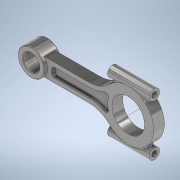
# Autodesk Inventor part: connecting_rod
Saved by Autodesk Inventor 2021 (Build 250183000, 183)
## iProperties
Created: 2020-11-10
Part Number: connecting_rod
Material: Сталь, высокопрочная, низколегированная
Document SubType Name: Modeling
Designer: panda
Density: 7.85 g/cm^3
Appearance: Сталь — полированная
Mass: 1160.23 g
Surface Area: 416.927 cm^2
Volume: 147.8 cm^3
Author: panda
Autodesk Inventor part; units mm, degrees
ref_plane "XZ Plane" through (0, 0, 0) normal (0, 1, 0) x (-1, 0, 0)
ref_plane "XY Plane" through (0, 0, 0) normal (0, 0, 1) x (1, 0, 0)
sketch "Эскиз1" plane through (0, 0, 0) normal (0, 0, 1) x (1, 0, 0)
  circle A0 centre (0, 0) radius 14
  circle A1 centre (0, 0) radius 22.5
  circle A2 centre (159, 0) radius 27.5
  arc A3 (128.2466, -30.0538) -> (128.2466, 30.0538) centre (159, 0) ccw
  line L0 (0, 14) -> (0, 15)
  line L1 (16.7705, 15) -> (92.4868, 15)
  line L2 (-29.6074, 0) -> (209.3399, 0) construction
  line L3 (16.7705, -15) -> (92.4868, -15)
  arc A4 (92.4868, 15) -> (128.2466, 30.0538) centre (92.4868, 65) ccw
  arc A5 (128.2466, -30.0538) -> (92.4868, -15) centre (92.4868, -65) ccw
  point P0 (118.7011, 15)
  point P1 (118.7011, -15)
  dimension "d0" = 28
  dimension "d1" = 45
  dimension "d2" = 159
  dimension "d3" = 55
  dimension "d4" = 86
  dimension "d5" = 15
  dimension "d6" = 50
  constraints: 8 end point, 8 point on circle, 4 centre point, 4 tangent, 3 coincident, 2 point on line, 2 symmetric about line, 1 equal radius, 1 horizontal, 1 perpendicular, 1 vertical, 1 vertical alignment, 5 other
  measures "d2" distance of point (0, 0) A2.centre
  measures "d3" diameter of A2
  measures "d4" diameter of A3
  measures "d5" distance of point (0, 0) L0.end
  measures "d6" radius of A4
extrude "Выдавливание1" add sketch "Эскиз1" against normal mid plane 18 contours A1 L1 A4 A3 A5 L3
extrude "Выдавливание2" add sketch "Эскиз1" along normal mid plane 28 contours A1
sketch "Эскиз2" plane through (0, 0, 9) normal (0, 0, 1) x (1, 0, 0)
  arc A0 (128.2466, -30.0538) -> (128.2466, 30.0538) centre (159, 0) ccw projected
  arc A1 (92.4868, 15) -> (128.2466, 30.0538) centre (92.4868, 65) ccw projected
  arc A2 (128.2466, -30.0538) -> (92.4868, -15) centre (92.4868, -65) ccw projected
  line L0 (16.7705, 15) -> (92.4868, 15) projected
  arc A3 (16.7705, -15) -> (16.7705, 15) centre (0, 0) ccw projected
  line L1 (16.7705, -15) -> (92.4868, -15)
  arc A4 (159, 43) -> (128.2466, 30.0538) centre (159, 0) ccw
  arc A5 (128.2466, -30.0538) -> (159, -43) centre (159, 0) ccw
  line L2 (159, -35) -> (159, -35.5)
  arc A6 (128.2466, -30.0538) -> (159, -43) centre (159, 0) ccw
  arc A7 (159, 43) -> (128.2466, 30.0538) centre (159, 0) ccw
  arc A8 (118.915, -13.371) -> (92.4868, -7) centre (92.4868, -65) ccw
  line L3 (92.4868, -7) -> (34.3693, -7)
  arc A9 (30.3845, -2.6522) -> (30.3845, 2.6522) centre (0, 0) ccw
  line L4 (34.3693, 7) -> (92.4868, 7)
  arc A10 (92.4868, 7) -> (118.915, 13.371) centre (92.4868, 65) ccw
  arc A11 (124.6123, 8.817) -> (124.6123, -8.817) centre (159, 0) ccw
  arc A12 (34.3693, 7) -> (30.3845, 2.6522) centre (34.3693, 3) ccw
  arc A13 (30.3845, -2.6522) -> (34.3693, -7) centre (34.3693, -3) ccw
  arc A14 (124.6123, 8.817) -> (118.915, 13.371) centre (120.7377, 9.8104) ccw
  arc A15 (118.915, -13.371) -> (124.6123, -8.817) centre (120.7377, -9.8104) ccw
  point P0 (29.6859, -7)
  point P1 (29.6859, 7)
  dimension "d11" = 8
  dimension "d12" = 71
  dimension "d13" = 4
  constraints: 30 point on circle, 12 centre point, 9 tangent, 8 end point, 3 equal radius, 2 coincident, 2 point on line, 1 horizontal, 1 vertical, 2 other
  measures "d11" radial gap between concentric circles of A1 A10
  measures "d12" diameter of A11
  measures "d13" radius of A12
extrude "Выдавливание3" cut sketch "Эскиз2" against normal blind 5 contours A8 L3 A13 A9 A12 L4 A10 A14 A11 A15
mirror "Зеркальное отражение1" about plane through (0, 0, 0) normal (0, 0, 1) of "Выдавливание3"
ref_plane "РабПлоскость1" through (159, 0, 0) normal (1, 0, 0) x (0, 1, 0)
sketch "Эскиз3" plane through (159, 0, 0) normal (1, 0, 0) x (0, 1, 0)
  line L0 (43, 9) -> (43, -9) projected
  circle A0 centre (43, 0) radius 9
  point P0 (0, 0)
  constraints: 1 centre point, 1 midpoint
extrude "Выдавливание4" add sketch "Эскиз3" along normal mid plane 70
sketch "Эскиз4" plane through (124, 43, 0) normal (-1, 0, 0) x (0, 0, 1)
  point P0 (0, -43)
  point P1 (0, 0)
hole "Отверстие1" at (124, 43, 0) direction (1, 0, 0) diameter 9 end through all
fillet "Сопряжение1" radius 2 2 edges at (185.3247, 34.0001, 0.0483) (132.6753, 34.0001, 0.0483)
mirror "Зеркальное отражение2" about plane through (0, 0, 0) normal (0, 1, 0) of "Выдавливание4", "Отверстие1", "Сопряжение1"
fillet "Сопряжение2" radius 1 24 edges at (63.4281, -7, 9) (31.4205, -5.7027, 9) (30.5, 0, 9) (31.4205, 5.7027, 9) (63.4281, 7, 9) (106.0795, 8.6152, 9) (123.2352, 12.9349, 9) (123.5, 0, 9) (123.2352, -12.9349, 9) (106.0795, -8.6152, 9) (-22.5, 0, 14) (-14, 0, 14) (123.2352, -12.9349, -9) (123.5, 0, -9) (123.2352, 12.9349, -9) (106.0795, 8.6152, -9) (63.4281, 7, -9) (31.4205, 5.7027, -9) (30.5, 0, -9) (31.4205, -5.7027, -9) (63.4281, -7, -9) (106.0795, -8.6152, -9) (-14, 0, -14) (-22.5, 0, -14)
